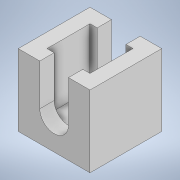
# Autodesk Inventor part: snapfit_v06
Saved by Autodesk Inventor 2022 (Build 260153000, 153)
## iProperties
Created: 2022-03-20
Part Number: snapfit_v06
Material: Generic
Document SubType Name: Modeling
Designer: LIMlab
Density: 1 g/cm^3
Appearance: Default
Author: LIMlab
Autodesk Inventor part; units mm, degrees
ref_plane "YZ Plane" through (0, 0, 0) normal (1, 0, 0) x (0, 1, 0)
ref_plane "XZ Plane" through (0, 0, 0) normal (0, 1, 0) x (-1, 0, 0)
ref_plane "XY Plane" through (0, 0, 0) normal (0, 0, 1) x (1, 0, 0)
sketch "Sketch1" plane through (0, 0, 0) normal (0, 1, 0) x (-1, 0, 0)
  line L0 (-2.5, 2.5) -> (2.5, 2.5)
  line L1 (2.5, 2.5) -> (2.5, -2.5)
  line L2 (2.5, -2.5) -> (-2.5, -2.5)
  line L3 (-2.5, -2.5) -> (-2.5, 2.5)
  line L4 (-2.5, 2.5) -> (2.5, -2.5) construction
  line L5 (2.5, 2.5) -> (-2.5, -2.5) construction
  point P0 (0, 0)
  dimension "d0" = 5
  dimension "d1" = 5
  constraints: 12 end point, 2 midpoint, 2 parallel, 1 horizontal, 1 perpendicular
  measures "d0" distance of L0.end L1.end
  measures "d1" distance of L1.end L2.end
extrude "Extrusion1" add sketch "Sketch1" along normal blind 5
shell "Shell1" thickness 1 removed faces 1 at (-0.8333, 5, -0.8333)
sketch "Sketch3" plane through (-2.5, 0, 2.5) normal (0, 0, 1) x (1, 0, 0)
  line L0 (2.5, 9.1674) -> (2.5, 2.1156) construction
  line L1 (1.4995, 9.1674) -> (1.4995, 2.1156)
  line L2 (3.5005, 2.1156) -> (3.5005, 9.1674)
  arc A0 (3.5005, 9.1674) -> (1.4995, 9.1674) centre (2.5, 9.1674) ccw
  arc A1 (1.4995, 2.1156) -> (3.5005, 2.1156) centre (2.5, 2.1156) ccw
  point P0 (2.5, 0)
  point P1 (2.5, 5.6415)
  constraints: 8 end point, 4 point on circle, 4 tangent, 2 centre point, 1 midpoint, 1 parallel, 1 vertical
extrude "Extrusion3" cut sketch "Sketch3" against normal through all
body "Solid1"
